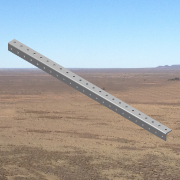
# Autodesk Inventor part: frame_angle_horiz
Saved by Autodesk Inventor 2014 SP1 (Build 180222100, 222)
## iProperties
Created: 2014-05-23
Part Number: frame_angle_horiz
Material: Steel, Mild
Document SubType Name: Modeling
Designer: Dave
Mass: 686.219 g
Surface Area: 605.745 cm^2
Volume: 87.3052 cm^3
Density: 7.86 g/cm^3
Appearance: Steel
Author: Dave
Autodesk Inventor part; units mm, degrees
ref_plane "YZ Plane" through (0, 0, 0) normal (1, 0, 0) x (0, 1, 0)
ref_plane "XZ Plane" through (0, 0, 0) normal (0, 1, 0) x (-1, 0, 0)
ref_plane "XY Plane" through (0, 0, 0) normal (0, 0, 1) x (1, 0, 0)
sketch "Sketch1" plane through (0, 0, 0) normal (1, 0, 0) x (0, 1, 0)
  line L0 (0, 0) -> (22.225, 0)
  line L1 (25.4, -3.175) -> (25.4, -25.4)
  line L2 (22.2268, -25.4) -> (22.2268, -6.3482)
  line L3 (19.0518, -3.1732) -> (0, -3.1732)
  line L4 (25.4, -25.4) -> (22.2268, -25.4)
  line L5 (0, 0) -> (0, -3.1732)
  arc A0 (25.4, -3.175) -> (22.225, 0) centre (22.225, -3.175) ccw
  arc A1 (22.2268, -6.3482) -> (19.0518, -3.1732) centre (19.0518, -6.3482) ccw
  point P0 (25.4, 0)
  dimension "d0" = 25.4
  dimension "d1" = 25.4
  dimension "d2" = 3.175
  constraints: 12 end point, 4 point on circle, 4 tangent, 3 perpendicular, 2 centre point, 2 point on line, 1 equal radius, 1 horizontal, 1 parallel, 1 other
  measures "d0" distance of L0.start point (25.4, 0)
  measures "d1" distance of point (25.4, 0) L1.end
  measures "d2" radius of A0
extrude "Extrusion1" add sketch "Sketch1" along normal blind 609.6
sketch "Sketch2" plane through (0, 0, 0) normal (0, 0, 1) x (1, 0, 0)
  line L0 (0, 0) -> (0, 22.225) projected
  circle A0 centre (12.7, 11.1125) radius 1.9225
  dimension "d5" = 12.7
  constraints: 1 centre point
  measures "d5" distance from line of A0.centre L0
hole "Hole1" at (12.7, 11.1125, 0) direction (0, 0, -1) diameter 6.35 end through all
pattern_linear "Rectangular Pattern1" count 24 spacing 25.4 along (1, 0, 0) of "Hole1"
sketch "Sketch3" plane through (0, 25.4, -3.175) normal (0, 1, 0) x (1, 0, 0)
  line L0 (0, 0) -> (0, 22.225) projected
  circle A0 centre (12.7, 11.1125) radius 5.2364
  point P0 (0, -3.175)
  dimension "d16" = 12.7
  constraints: 1 centre point
  measures "d16" distance from line of A0.centre L0
hole "Hole2" at (12.7, 25.4, -14.2875) direction (0, -1, 0) diameter 6.35 end through all
pattern_linear "Rectangular Pattern2" count 24 spacing 25.4 along (1, 0, 0) of "Hole2"
body "Solid1"
